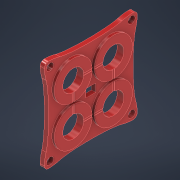
# Autodesk Inventor part: BatteryRoof
Saved by Autodesk Inventor 2022 (Build 260153000, 153)
## iProperties
Created: 2022-04-11
Part Number: BatteryRoof
Material: ABS Plastic
Document SubType Name: Modeling
Designer: ForseFire
Density: 1.06 g/cm^3
Appearance: Red
Author: ForseFire
Autodesk Inventor part; units mm, degrees
ref_plane "YZ Plane" through (0, 0, 0) normal (1, 0, 0) x (0, 1, 0)
ref_plane "XZ Plane" through (0, 0, 0) normal (0, 1, 0) x (-1, 0, 0)
ref_plane "XY Plane" through (0, 0, 0) normal (0, 0, 1) x (1, 0, 0)
sketch "Sketch1" plane through (0, 0, 0) normal (1, 0, 0) x (0, 1, 0)
  line L0 (-22, -22) -> (22, -22)
  line L1 (22, -22) -> (22, 22)
  line L2 (22, 22) -> (-22, 22)
  line L3 (-22, 22) -> (-22, -22)
  line L4 (-22, -22) -> (22, 22) construction
  line L5 (22, -22) -> (-22, 22) construction
  line L6 (-19.3, -19.3) -> (19.3, -19.3)
  line L7 (19.3, -19.3) -> (19.3, 19.3)
  line L8 (19.3, 19.3) -> (-19.3, 19.3)
  line L9 (-19.3, 19.3) -> (-19.3, -19.3)
  line L10 (-19.3, -19.3) -> (19.3, 19.3) construction
  line L11 (19.3, -19.3) -> (-19.3, 19.3) construction
  circle A0 centre (19.3, 19.3) radius 1.7
  circle A1 centre (19.3, -19.3) radius 1.7
  circle A2 centre (-19.3, -19.3) radius 1.7
  circle A3 centre (-19.3, 19.3) radius 1.7
  line L12 (19.3, 0) -> (0, 0)
  circle A4 centre (9.5, -9.5) radius 5
  circle A5 centre (9.5, 9.5) radius 5
  line L13 (0, 0) -> (-19.3, 0)
  circle A6 centre (-9.5, -9.5) radius 5
  circle A7 centre (-9.5, 9.5) radius 5
  circle A8 centre (9.5, -9.5) radius 9.5
  circle A9 centre (9.5, 9.5) radius 9.5
  circle A10 centre (-9.5, 9.5) radius 9.5
  circle A11 centre (-9.5, -9.5) radius 9.5
  point P0 (0, 0)
  point P1 (0, 0)
  point P2 (6.364, 6.364)
  dimension "d0" = 44
  dimension "d1" = 44
  dimension "d6" = 38.6
  dimension "d7" = 38.6
  dimension "d8" = 3.4
  dimension "d9" = 3.4
  dimension "d10" = 3.4
  dimension "d11" = 3.4
  dimension "d19" = 10
  dimension "d20" = 10
  dimension "d21" = 10
  dimension "d22" = 10
  dimension "d23" = 19
  dimension "d24" = 19
  dimension "d25" = 19
  dimension "d26" = 19
  constraints: 28 end point, 12 centre point, 8 coincident, 8 midpoint, 5 point on line, 4 parallel, 3 equal radius, 2 horizontal, 2 perpendicular, 1 vertical alignment
  measures "d0" distance of L2.end L1.end
  measures "d1" distance of L0.end L1.end
  measures "d6" distance of L8.end L7.end
  measures "d7" distance of L6.end L7.end
  measures "d8" diameter of A0
  measures "d9" diameter of A1
  measures "d10" diameter of A2
  measures "d11" diameter of A3
  measures "d19" diameter of A4
  measures "d20" diameter of A5
  measures "d21" diameter of A6
  measures "d22" diameter of A7
  measures "d23" diameter of A8
  measures "d24" diameter of A9
  measures "d25" diameter of A10
  measures "d26" diameter of A11
extrude "Extrusion1" add sketch "Sketch1" along normal blind 2 contours L3 L2 L1 L0 | A2 L9 L13 A11 A8 L12 L7 A1 L6 | L9 A3 L8 A0 L7 L12 A9 A10 L13 | A10 A9 L12 L13 | A10 | L13 L12 A8 A11 | A11 | A9 | A8
fillet "Fillet1" radius 2 4 edges at (1, -22, 22) (1, -22, -22) (1, 22, -22) (1, 22, 22)
sketch "Sketch2" plane through (2, 0, 0) normal (1, 0, 0) x (0, 0, -1)
  arc A0 (-20, 22) -> (-22, 20) centre (-20, 20) ccw projected
  line L0 (-22, 20) -> (-22, -20) projected
  arc A1 (-22, -20) -> (-20, -22) centre (-20, -20) ccw projected
  line L1 (-20, -22) -> (20, -22) projected
  arc A2 (20, -22) -> (22, -20) centre (20, -20) ccw projected
  line L2 (22, -20) -> (22, 20) projected
  arc A3 (22, 20) -> (20, 22) centre (20, 20) ccw projected
  line L3 (20, 22) -> (-20, 22) projected
  circle A4 centre (-19.3, -19.3) radius 1.7 projected
  circle A5 centre (19.3, -19.3) radius 1.7 projected
  circle A6 centre (9.5, 9.5) radius 5 projected
  circle A7 centre (9.5, -9.5) radius 5 projected
  circle A8 centre (19.3, 19.3) radius 1.7 projected
  circle A9 centre (-9.5, 9.5) radius 5 projected
  circle A10 centre (-9.5, -9.5) radius 5 projected
  circle A11 centre (-19.3, 19.3) radius 1.7 projected
  circle A12 centre (-9.5, -9.5) radius 9
  circle A13 centre (-9.5, 9.5) radius 9
  circle A14 centre (9.5, 9.5) radius 9
  circle A15 centre (9.5, -9.5) radius 9
  point P0 (0, 0)
  dimension "d27" = 18
  dimension "d28" = 18
  dimension "d29" = 18
  dimension "d30" = 18
  constraints: 4 centre point, 4 coincident
  measures "d27" diameter of A12
  measures "d28" diameter of A13
  measures "d29" diameter of A14
  measures "d30" diameter of A15
extrude "Extrusion2" add sketch "Sketch2" along normal blind 1.2 contours A12 | A13 | A14 | A15
sketch "Sketch4" plane through (0, 0, 0) normal (-1, 0, 0) x (0, 0, 1)
  circle A0 centre (0, 0) radius 2.5
  line L0 (2.3, -1.95) -> (-2.3, -1.95)
  line L1 (-2.3, -1.95) -> (-2.3, 1.95)
  line L2 (-2.3, 1.95) -> (2.3, 1.95)
  line L3 (2.3, 1.95) -> (2.3, -1.95)
  line L4 (2.3, -1.95) -> (-2.3, 1.95) construction
  line L5 (-2.3, -1.95) -> (2.3, 1.95) construction
  dimension "d36" = 5
  dimension "d50" = 4.6
  dimension "d51" = 3.9
  constraints: 12 end point, 2 midpoint, 2 parallel, 1 centre point, 1 coincident, 1 horizontal, 1 perpendicular
  measures "d36" diameter of A0
  measures "d50" distance of L1.end L2.end
  measures "d51" distance of L0.end L1.end
extrude "Extrusion4" cut sketch "Sketch4" against normal blind 2 contours L3 A0 L0 L1 L2 | A0 L2 L3 | L3 L0 A0 | A0 L1 L2 | L0 L1 A0
sketch "Sketch5" plane through (0, 0, 0) normal (-1, 0, 0) x (0, 0, 1)
  line L0 (20, -22) -> (-20, -22) projected
  ellipse E0 centre (0, -22) end of major axis (-16, -22) minor radius 2
  ellipse E1 centre (21.9865, 0) end of major axis (21.9865, -16) minor radius 2
  line L1 (-20, 22) -> (20, 22) projected
  ellipse E2 centre (0, 22) end of major axis (-16, 22) minor radius 2
  line L2 (-22, -20) -> (-22, 20) projected
  ellipse E3 centre (-22, 0) end of major axis (-22, 16) minor radius 2
  point P0 (0, 0)
  dimension "d39" = 2
  dimension "d40" = 16
  dimension "d41" = 2
  dimension "d42" = 16
  dimension "d43" = 2
  dimension "d44" = 16
  dimension "d45" = 2
  dimension "d46" = 16
  constraints: 3 midpoint, 8 other
extrude "Extrusion5" cut sketch "Sketch5" against normal blind 2
fillet "Fillet2" radius 20 8 edges at (1, -22, -16) (1, -16, -22) (1, 16, -22) (1, 22, -16) (1, 22, 16) (1, 15.9996, 22) (1, -15.9996, 22) (1, -22, 16)
sketch "Sketch6" plane through (3.2, 9.5, -9.5) normal (1, 0, 0) x (0, 0, -1)
  circle A0 centre (0, 0) radius 9 projected
  circle A1 centre (0, 0) radius 5 projected
  circle A2 centre (-19, 0) radius 9 projected
  circle A3 centre (-19, 0) radius 5 projected
  circle A4 centre (0, -19) radius 9 projected
  circle A5 centre (0, -19) radius 5 projected
  circle A6 centre (-19, -19) radius 9 projected
  circle A7 centre (-19, -19) radius 5 projected
  line L0 (-14.1, 0.457) -> (-4.9, 0.457)
  line L1 (-4.9, 0.457) -> (-4.9, -0.543)
  line L2 (-4.9, -0.543) -> (-14.1, -0.543)
  line L3 (-14.1, -0.543) -> (-14.1, 0.457)
  line L4 (-14.1, 0.457) -> (-4.9, -0.543) construction
  line L5 (-4.9, 0.457) -> (-14.1, -0.543) construction
  line L6 (0.5, -4.9) -> (-0.5, -4.9)
  line L7 (-0.5, -4.9) -> (-0.5, -14.1)
  line L8 (-0.5, -14.1) -> (0.5, -14.1)
  line L9 (0.5, -14.1) -> (0.5, -4.9)
  line L10 (0.5, -4.9) -> (-0.5, -14.1) construction
  line L11 (-0.5, -4.9) -> (0.5, -14.1) construction
  line L12 (-4.9, -19.5) -> (-14.1, -19.5)
  line L13 (-14.1, -19.5) -> (-14.1, -18.5)
  line L14 (-14.1, -18.5) -> (-4.9, -18.5)
  line L15 (-4.9, -18.5) -> (-4.9, -19.5)
  line L16 (-4.9, -19.5) -> (-14.1, -18.5) construction
  line L17 (-14.1, -19.5) -> (-4.9, -18.5) construction
  line L18 (-18.5, -14.1) -> (-19.5, -14.1)
  line L19 (-19.5, -14.1) -> (-19.5, -4.9)
  line L20 (-19.5, -4.9) -> (-18.5, -4.9)
  line L21 (-18.5, -4.9) -> (-18.5, -14.1)
  line L22 (-18.5, -14.1) -> (-19.5, -4.9) construction
  line L23 (-19.5, -14.1) -> (-18.5, -4.9) construction
  point P0 (-9.5, -9.5)
  point P1 (-9.5, -0.043)
  point P2 (0, -9.5)
  point P3 (-9.5, -19)
  point P4 (-19, -9.5)
  dimension "d52" = 9.2
  dimension "d53" = 1
  dimension "d54" = 1
  dimension "d55" = 9.2
  dimension "d56" = 9.2
  dimension "d57" = 1
  dimension "d58" = 1
  dimension "d59" = 9.2
  constraints: 48 end point, 8 midpoint, 8 parallel, 4 horizontal, 4 perpendicular
  measures "d52" distance of L1.end L2.end
  measures "d53" distance between parallel lines of L2 L0
  measures "d54" distance of L8.end L7.end
  measures "d55" distance of L7.end L6.end
  measures "d56" distance of L13.end L14.end
  measures "d57" distance of L12.end L13.end
  measures "d58" distance of L19.end L20.end
  measures "d59" distance of L18.end L19.end
extrude "Extrusion6" cut sketch "Sketch6" against normal blind 0.2 contours L0 A1 L2 A0 | A0 L2 A2 L0 | L9 A4 L7 A0 | A0 L7 A1 L9 | A2 L2 A3 L0 | L0 L1 L2 A1 | L9 A5 L7 A4 | A1 L7 L6 L9 | L19 A3 L21 A2 | A2 L21 A6 L19 | A3 L2 L3 L0 | L9 L8 L7 A5 | A6 L21 A7 L19 | L19 L20 L21 A3 | L14 A5 L12 A4 | A4 L12 A6 L14 | L12 A7 L14 A6 | A7 L21 L18 L19 | L14 L15 L12 A5 | L12 L13 L14 A7
body "Solid1"
